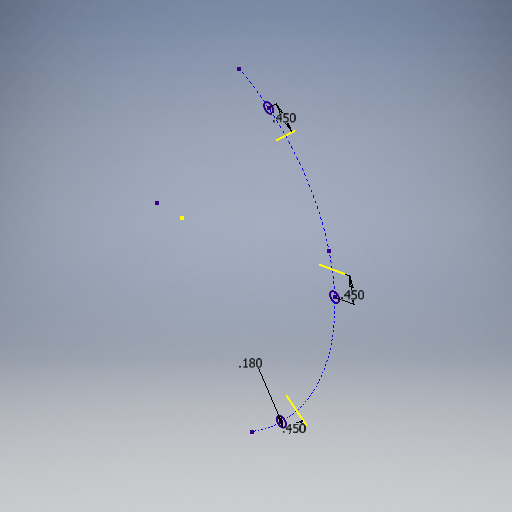
# Autodesk Inventor part: Robert
Saved by Autodesk Inventor 2026.1 (Build 301233000, 233)
## iProperties
Created: 2025-10-13
Part Number: Robert
Material: Plastic, Opaque Black
Document SubType Name: Modeling
Designer: Teddy
Density: 0.952 g/cm^3
Appearance: Smooth - Black
Author: Teddy
Autodesk Inventor part; units mm, degrees
ref_plane "YZ Plane" through (0, 0, 0) normal (1, 0, 0) x (0, 1, 0)
ref_plane "XZ Plane" through (0, 0, 0) normal (0, 1, 0) x (-1, 0, 0)
ref_plane "XY Plane" through (0, 0, 0) normal (0, 0, 1) x (1, 0, 0)
ref_plane "Work Plane1" through (0, 0, 0) normal (0, 0, 1) x (1, 0, 0)
sketch "Sketch1" plane through (0, 0, 0) normal (0, 0, 1) x (1, 0, 0)
  circle A0 centre (33.02, 0) radius 2.286 projected
  circle A1 centre (0, 20.32) radius 2.286 projected
  circle A2 centre (0, -20.32) radius 2.286 projected
  circle A3 centre (-33.02, 0) radius 2.286 projected
  circle A4 centre (-33.02, 0) radius 2.286 projected
  circle A5 centre (33.02, 0) radius 2.286 projected
  circle A6 centre (0, 20.32) radius 2.286 projected
  circle A7 centre (0, -20.32) radius 2.286 projected
  arc A8 (26.3675, -11.6445) -> (27.8119, -10.2) centre (26.3675, -10.2) ccw projected
  line L0 (26.3675, -11.6445) -> (25.45, -11.6445) projected
  arc A9 (25.45, -11.6445) -> (23.5945, -13.5) centre (25.45, -13.5) ccw projected
  line L1 (23.5945, -13.5) -> (23.5945, -14.2175) projected
  arc A10 (22.452, -15.63) -> (23.5945, -14.2175) centre (22.15, -14.2175) ccw projected
  line L2 (22.452, -15.63) -> (22.452, -15.827) projected
  line L3 (22.452, -15.827) -> (21.448, -15.827) projected
  line L4 (21.448, -15.827) -> (21.448, -15.6619) projected
  line L5 (21.448, -15.6619) -> (-22.15, -15.6619) projected
  arc A11 (-23.5945, -14.2175) -> (-22.15, -15.6619) centre (-22.15, -14.2175) ccw projected
  line L6 (-23.5945, -14.2175) -> (-23.5945, -13.5) projected
  arc A12 (-23.5945, -13.5) -> (-25.45, -11.6445) centre (-25.45, -13.5) ccw projected
  line L7 (-25.45, -11.6445) -> (-26.3675, -11.6445) projected
  arc A13 (-27.8119, -10.2) -> (-26.3675, -11.6445) centre (-26.3675, -10.2) ccw projected
  line L8 (-27.8119, -10.2) -> (-27.8119, 10.2) projected
  arc A14 (-26.3675, 11.6445) -> (-27.8119, 10.2) centre (-26.3675, 10.2) ccw projected
  line L9 (-26.3675, 11.6445) -> (-25.45, 11.6445) projected
  arc A15 (-25.45, 11.6445) -> (-23.5945, 13.5) centre (-25.45, 13.5) ccw projected
  line L10 (-23.5945, 13.5) -> (-23.5945, 14.2175) projected
  arc A16 (-22.15, 15.6619) -> (-23.5945, 14.2175) centre (-22.15, 14.2175) ccw projected
  line L11 (-22.15, 15.6619) -> (21.448, 15.6619) projected
  line L12 (21.448, 15.6619) -> (21.448, 15.827) projected
  line L13 (21.448, 15.827) -> (22.452, 15.827) projected
  line L14 (22.452, 15.827) -> (22.452, 15.63) projected
  arc A17 (23.5945, 14.2175) -> (22.452, 15.63) centre (22.15, 14.2175) ccw projected
  line L15 (23.5945, 14.2175) -> (23.5945, 13.5) projected
  arc A18 (23.5945, 13.5) -> (25.45, 11.6445) centre (25.45, 13.5) ccw projected
  line L16 (25.45, 11.6445) -> (26.3675, 11.6445) projected
  arc A19 (27.8119, 10.2) -> (26.3675, 11.6445) centre (26.3675, 10.2) ccw projected
  line L17 (27.8119, 10.2) -> (27.8119, -10.2) projected
  arc A20 (26.4301, -16.225) -> (27.7187, -15.3162) centre (25.05, -12.9) ccw projected
  line L18 (27.7187, -15.3162) -> (37.7272, -4.262) projected
  arc A21 (37.7272, -4.262) -> (37.7272, 4.262) centre (33.02, 0) ccw projected
  line L19 (37.7272, 4.262) -> (27.7187, 15.3162) projected
  arc A22 (27.7187, 15.3162) -> (26.4301, 16.225) centre (25.05, 12.9) ccw projected
  line L20 (26.4301, 16.225) -> (2.4343, 26.1849) projected
  arc A23 (2.4343, 26.1849) -> (-2.4343, 26.1849) centre (0, 20.32) ccw projected
  line L21 (-2.4343, 26.1849) -> (-26.4301, 16.225) projected
  arc A24 (-26.4301, 16.225) -> (-27.7187, 15.3162) centre (-25.05, 12.9) ccw projected
  line L22 (-27.7187, 15.3162) -> (-37.7272, 4.262) projected
  arc A25 (-37.7272, 4.262) -> (-37.7272, -4.262) centre (-33.02, 0) ccw projected
  line L23 (-37.7272, -4.262) -> (-27.7187, -15.3162) projected
  arc A26 (-27.7187, -15.3162) -> (-26.4301, -16.225) centre (-25.05, -12.9) ccw projected
  line L24 (-26.4301, -16.225) -> (-2.4343, -26.1849) projected
  arc A27 (-2.4343, -26.1849) -> (2.4343, -26.1849) centre (0, -20.32) ccw projected
  line L25 (2.4343, -26.1849) -> (26.4301, -16.225) projected
  circle A28 centre (28.3975, 78.8302) radius 3.9624 construction
  circle A29 centre (56.9076, 55.2992) radius 3.9624 construction
  circle A30 centre (73.3819, 22.2064) radius 3.9624 construction
  circle A31 centre (74.9718, -14.7261) radius 3.9624 construction
  circle A32 centre (61.4026, -49.1123) radius 3.9624 construction
  circle A33 centre (35.0203, -75.0066) radius 3.9624 construction
  circle A34 centre (-62.1863, 61.5138) radius 2.1844 projected
  circle A35 centre (-72.7933, -46.4423) radius 2.1844 projected
  arc A36 (35.0203, -75.0066) -> (28.3975, 78.8302) centre (-12.7, 0) ccw construction
  arc A37 (38.4289, -80.3642) -> (31.333, 84.461) centre (-12.7, 0) ccw
  arc A38 (31.6117, -69.649) -> (25.4619, 73.1995) centre (-12.7, 0) ccw
  arc A39 (31.6117, -69.649) -> (38.4289, -80.3642) centre (35.0203, -75.0066) ccw
  arc A40 (31.333, 84.461) -> (25.4619, 73.1995) centre (28.3975, 78.8302) ccw
  circle A41 centre (28.3975, 78.8302) radius 2.286
  circle A42 centre (56.9076, 55.2992) radius 2.286
  circle A43 centre (73.3819, 22.2064) radius 2.286
  circle A44 centre (74.9718, -14.7261) radius 2.286
  circle A45 centre (61.4026, -49.1123) radius 2.286
  circle A46 centre (35.0203, -75.0066) radius 2.286
  arc A47 (39.7923, -82.5072) -> (32.5072, 86.7133) centre (-12.7, 0) ccw construction
  circle A48 centre (32.5072, 86.7133) radius 2.286
  circle A49 centre (63.8683, 60.8291) radius 2.286
  circle A50 centre (81.9901, 24.427) radius 2.286
  circle A51 centre (83.739, -16.1987) radius 2.286
  circle A52 centre (68.8128, -54.0236) radius 2.286
  circle A53 centre (39.7923, -82.5072) radius 2.286
  line L26 (28.3975, 78.8302) -> (32.5072, 86.7133) construction
  arc A54 (40.0791, 79.2901) -> (25.4619, 73.1995) centre (30.2292, 82.3438) ccw
  arc A55 (64.5022, 55.7888) -> (59.1019, 62.5863) centre (63.8683, 60.8291) ccw
  arc A56 (56.9737, 64.9472) -> (60.6061, 64.7232) centre (58.908, 66.7503) ccw
  arc A57 (66.9239, 56.7708) -> (66.3206, 53.1818) centre (68.5145, 54.6582) ccw
  arc A58 (77.3665, 30.9934) -> (80.5938, 29.3113) centre (79.867, 31.8539) ccw
  arc A59 (80.519, 19.5646) -> (78.3505, 27.971) centre (81.9901, 24.427) ccw
  arc A60 (83.1308, 19.4767) -> (81.1199, 16.4434) centre (83.7246, 16.8999) ccw
  arc A61 (82.186, -8.3194) -> (84.4501, -11.1688) centre (84.8203, -8.5504) ccw
  arc A62 (80.4175, -20.0424) -> (81.8556, -11.4808) centre (83.739, -16.1987) ccw
  arc A63 (82.7677, -21.185) -> (79.6969, -23.1382) centre (82.2621, -23.7806) ccw
  arc A64 (70.5988, -46.1938) -> (71.5083, -49.7177) centre (72.9114, -47.4763) ccw
  arc A65 (64.2151, -56.1839) -> (69.0111, -48.9474) centre (68.8128, -54.0236) ccw
  arc A66 (65.8973, -58.1837) -> (62.2976, -58.719) centre (64.3797, -60.3492) ccw
  point P0 (0, 0)
  point P1 (70.5988, -46.1938)
  point P2 (62.2976, -58.719)
  point P3 (82.186, -8.3194)
  point P4 (79.6969, -23.1382)
  point P5 (77.3665, 30.9934)
  dimension "d0" = 12.7
  dimension "d3" = 4.572
  dimension "d4" = 4.572
  dimension "d5" = 4.572
  dimension "d6" = 4.572
  dimension "d7" = 4.572
  dimension "d8" = 4.572
  dimension "d26" = 8.89
  dimension "d29" = 120
  dimension "d32" = 5.08
  dimension "d35" = 72
  constraints: 55 point on circle, 31 centre point, 9 tangent, 8 coincident, 2 end point, 1 equal radius, 1 line through centre, 1 point on line, 50 other
  measures "d0" diameter of A39
  measures "d3" diameter of A41
  measures "d4" diameter of A42
  measures "d5" diameter of A43
  measures "d6" diameter of A44
  measures "d7" diameter of A45
  measures "d8" diameter of A46
  measures "d26" radial gap between concentric circles of A36 A47
  measures "d32" radius of A55
extrude "Extrusion1" add sketch "Sketch1" along normal blind 8.89 contours A39 A38 A40 A37 | A37 A65 A66 | A37 A65 | A54 A37 A40 | A37 A64 A65 | A56 A55 A37 | A37 A62 A63 | A55 A37 | A37 A62 | A55 A57 A37 | A37 A61 A62 | A58 A59 A37 | A37 A59 A60 | A59 A37 | A41 | A42 | A43 | A44 | A45 | A46
fillet "Fillet2" radius 3.175 1 edges at (40.0791, 79.2901, 4.445)
sketch "Sketch2" plane through (0, 0, 8.89) normal (0, 0, 1) x (1, 0, 0)
  arc A0 (31.6117, -69.649) -> (25.4619, 73.1995) centre (-12.7, 0) ccw projected
  arc A1 (38.4289, -80.3642) -> (62.2976, -58.719) centre (-12.7, 0) ccw projected
  line L0 (31.2583, 69.8725) -> (38.0211, 80.6221)
  line L1 (46.9952, 57.0174) -> (56.1791, 65.7893)
  line L2 (68.6393, 14.0864) -> (81.153, 16.2536)
  line L3 (69.6161, -6.2101) -> (82.2801, -7.1655)
  line L4 (52.1949, -51.0212) -> (62.1787, -58.8706)
  line L5 (37.7652, -65.3281) -> (45.5291, -75.3786)
  arc A2 (82.186, -8.3194) -> (81.1199, 16.4434) centre (-12.7, 0) ccw projected
  line L6 (38.0211, 80.6221) -> (40.3498, 84.3236)
  arc A3 (40.4666, 81.1022) -> (25.4619, 73.1995) centre (30.2292, 82.3438) ccw projected
  arc A4 (56.9737, 64.9472) -> (40.0791, 79.2901) centre (-12.7, 0) ccw projected
  arc A5 (40.4666, 81.1022) -> (41.8018, 78.116) centre (43.6185, 80.7199) ccw projected
  point P0 (0, 0)
  point P1 (37.7652, -65.3281)
  point P2 (45.5291, -75.3786)
  point P3 (62.1787, -58.8706)
  point P4 (52.1949, -51.0212)
  point P5 (69.6161, -6.2101)
  point P6 (82.2658, -7.3525)
  point P7 (81.1848, 16.0688)
  point P8 (68.6393, 14.0864)
  dimension "d10" = 20.32
  dimension "d14" = 96
  dimension "d38" = 7.5121
  constraints: 14 end point, 5 point on circle, 4 line through centre, 1 collinear, 13 other
  measures "d10" distance of L0.start L1.start
  measures "d38" distance from line of L0 A3.centre
extrude "Extrusion2" cut sketch "Sketch2" against normal blind 3.81 contours A0 L4 A1 L5 | A0 L2 A2 L3 | A0 L0 L6 A3 A5 A4 L1
sketch "Sketch3" plane through (0, 0, 5.08) normal (0, 0, 1) x (1, 0, 0)
  circle A0 centre (43.1588, 69.1592) radius 2.286
  circle A1 centre (76.1195, 3.7817) radius 2.286
  circle A2 centre (49.5422, -63.4753) radius 2.286
  arc A3 (35.0203, -75.0066) -> (28.3975, 78.8302) centre (-12.7, 0) ccw construction
  line L0 (56.1791, 65.7893) -> (46.9952, 57.0174) projected
  line L1 (68.6393, 14.0864) -> (81.153, 16.2536) projected
  line L2 (52.1949, -51.0212) -> (62.1787, -58.8706) projected
  point P0 (0, 0)
  point P1 (73.3819, 22.2064)
  dimension "d18" = 4.572
  dimension "d19" = 11.43
  dimension "d20" = 11.43
  dimension "d21" = 11.43
  constraints: 6 point on circle, 4 centre point, 2 equal radius
  measures "d18" diameter of A2
  measures "d19" distance from line of L0 A0.centre
  measures "d20" distance from line of A1.centre L1
  measures "d21" distance from line of L2 A2.centre
extrude "Extrusion3" cut sketch "Sketch3" against normal through all
fillet "Fillet1" radius 3.175 11 edges at (31.2583, 69.8725, 6.985) (56.1791, 65.7893, 6.985) (45.5291, -75.3786, 6.985) (37.7652, -65.3281, 6.985) (52.1949, -51.0212, 6.985) (62.1787, -58.8706, 6.985) (82.2801, -7.1655, 6.985) (69.6161, -6.2101, 6.985) (81.153, 16.2536, 6.985) (68.6393, 14.0864, 6.985) (46.9952, 57.0174, 6.985)
body "Solid1"
